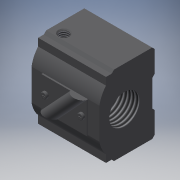
# Autodesk Inventor part: BNT 1605-2.6 Nut
Saved by Autodesk Inventor 2016 (Build 200138000, 138)
## iProperties
Category: PARTsolutions
Company: THK
Created: 2017-05-16
Part Number: BNT 1605-2.6 Nut
Catalog Web Link: www.cadenas.de
Description: BNT Nut-
Vendor: THK
Document SubType Name: Modeling
Designer: psAdmin
Manufacturer: THK
Mass: 33.6267 g
Surface Area: 94.5297 cm^2
Volume: 33.6267 cm^3
Density: 1 g/cm^3
Material: Generic
Appearance: PSOLRGB-192-192-192
PSOL_IDENT_0: {$CADENAS_DATA\23d-libs\thk\fed_screw\ball_screw\ball_screw\standard_lead_rbs\bnt\bnt_nut.prj},175 {
PSOL_IDENT_1: VTYP=3D},{NB=BNT 1605-2.6 Nut},{LINA=BNT 1605-2.6 Nut},{NN=BNT Nut},{DATE=08.03.2011 04:19:39},{GEOM
PSOL_IDENT_2: DATE=23.11.2007 13:11:00},{VERSION=},{LINEID=10},{LINESUBID=-1},{WBVAR=}  {NB=BNT 1605-2.6 Nut},{LIN
PSOL_IDENT_3: A=BNT 1605-2.6 Nut},{KT=DUMMY},{MN=BNT 1605-2.6},{L=36.000},{EL=1711.000},{W=42.000},{F=16.000},{B=3
PSOL_IDENT_4: 2.000},{C=22.000},{W1=21.000},{T=21.500},{M=32.500},{NDM=5.000},{KDM=4.134},{SL=8.000},{N1=6.000},{N
PSOL_IDENT_5: 2=2.000},{A=6.000},{M1=29.250},{X1=1.260},{X2=3.000},{R1=15.320},{X3=3.990},{ANG=47.0},{DK=3.200},{Y=
PSOL_IDENT_6: 0.740},{X4=0.300},{SD=16},{SL2=7.000},{Y2=11.700}
NN: BNT Nut
NB: BNT 1605-2.6 Nut
NBSYN: $MN. Nut
LINA: BNT 1605-2.6 Nut
MN: BNT 1605-2.6
L: 36.000
EL: 1711.000
W: 42.000
F: 16.000
B: 32.000
C: 22.000
W1: 21.000
T: 21.500
M: 32.500
NDM: 5.000
KDM: 4.134
SL: 8.000
N1: 6.000
N2: 2.000
A: 6.000
M1: 29.250
X1: 1.260
X2: 3.000
R1: 15.320
X3: 3.990
ANG: 47.0
DK: 3.200
Y: 0.740
X4: 0.300
SD: 16
SL2: 7.000
Y2: 11.700
SUPPLIER: THK
ARTICLENO: BNT 1605-2.6 Nut
BOMINFO: BNT 1605-2.6 Nut
CREATOR: CADENAS GmbH
Title: BNT 1605-2.6 Nut
Author: Cadenas PARTsolutions
Autodesk Inventor part; units mm, degrees
sketch "Sketch_1" plane through (0, 0, 0) normal (1, 0, 0) x (0, 1, 0)
  line L0 (14.74, 21) -> (-5.5, 21)
  line L1 (-5.5, 21) -> (-6.76, 19.74)
  line L2 (-6.76, 19.74) -> (-9.76, 19.74)
  line L3 (-9.76, 19.74) -> (-9.76, 15.75)
  arc A0 (-9.76, 15.75) -> (-13.25, 8.26) centre (1.867, 5.7743) ccw
  line L4 (-13.25, 8.26) -> (-13.25, -8.26)
  arc A1 (-13.25, -8.26) -> (-9.76, -15.75) centre (1.867, -5.7743) ccw
  line L5 (-9.76, -15.75) -> (-9.76, -19.74)
  line L6 (-9.76, -19.74) -> (-6.76, -19.74)
  line L7 (-6.76, -19.74) -> (-5.5, -21)
  line L8 (-5.5, -21) -> (14.74, -21)
  line L9 (14.74, -21) -> (16, -19.74)
  line L10 (16, -19.74) -> (16, -8.26)
  line L11 (16, -8.26) -> (14.74, -7)
  line L12 (14.74, -7) -> (14.74, 7)
  line L13 (14.74, 7) -> (16, 8.26)
  line L14 (16, 8.26) -> (16, 19.74)
  line L15 (16, 19.74) -> (14.74, 21)
  circle A2 centre (0, 0) radius 8
  constraints: 32 end point, 4 point on circle, 3 centre point
extrude "Extrusion1" add sketch "Sketch_1" along normal blind 36
sketch "Sketch_2" plane through (18, 0, 0) normal (0.682, 0, 0.7314) x (0.7314, 0, -0.682)
  line L0 (-18, -14.0625) -> (-3.1468, -14.0625)
  arc A0 (-3.1468, -14.0625) -> (3.1468, -14.0625) centre (0, -13.25) ccw
  line L1 (3.1468, -14.0625) -> (18, -14.0625)
  line L2 (18, -14.0625) -> (18, -13.25)
  line L3 (18, -13.25) -> (-18, -13.25)
  line L4 (-18, -13.25) -> (-18, -14.0625)
  constraints: 10 end point, 2 point on circle, 1 centre point
extrude "Extrusion2" add sketch "Sketch_2" along normal mid plane 36
sketch "Sketch_3" plane through (0, -13.25, 0) normal (0, 1, 0) x (1, 0, 0)
  line L0 (-18, -36) -> (54, -36)
  line L1 (54, -36) -> (54, 36)
  line L2 (54, 36) -> (-18, 36)
  line L3 (-18, 36) -> (-18, -36)
  line L4 (6, -8.26) -> (30, -8.26)
  line L5 (30, -8.26) -> (30, 8.26)
  line L6 (30, 8.26) -> (6, 8.26)
  line L7 (6, 8.26) -> (6, -8.26)
  constraints: 16 end point
extrude "Extrusion3" cut sketch "Sketch_3" against normal blind 3.25
sketch "Sketch_4" plane through (0, 0, 0) normal (0, 0, 1) x (1, 0, 0)
  line L0 (8.34, -15.3425) -> (8.34, -14.0625)
  line L1 (8.34, -14.0625) -> (9.94, -14.0625)
  line L2 (9.94, -14.0625) -> (9.94, -15.0225)
  arc A0 (9.62, -15.3425) -> (9.94, -15.0225) centre (9.62, -15.0225) ccw
  line L3 (9.62, -15.3425) -> (8.34, -15.3425)
  line L4 (8.34, -15.3425) -> (8.34, -14.0625)
  constraints: 10 end point, 2 point on circle, 1 centre point
revolve "Revolution1" add sketch "Sketch_4" angle 360 about axis through (8.34, -15.3425, 0) along (0, -1, 0)
sketch "Sketch_5" plane through (0, 0, 0) normal (0, 0, 1) x (1, 0, 0)
  line L0 (27.66, -15.3425) -> (27.66, -14.0625)
  line L1 (27.66, -14.0625) -> (29.26, -14.0625)
  line L2 (29.26, -14.0625) -> (29.26, -15.0225)
  arc A0 (28.94, -15.3425) -> (29.26, -15.0225) centre (28.94, -15.0225) ccw
  line L3 (28.94, -15.3425) -> (27.66, -15.3425)
  line L4 (27.66, -15.3425) -> (27.66, -14.0625)
  constraints: 10 end point, 2 point on circle, 1 centre point
revolve "Revolution2" add sketch "Sketch_5" angle 360 about axis through (27.66, -15.3425, 0) along (0, -1, 0)
sketch "Sketch_6" plane through (0, -15.3425, 0) normal (0, 1, 0) x (1, 0, 0)
  line L0 (26.86, 0.15) -> (26.86, -0.15)
  line L1 (26.86, -0.15) -> (27.51, -0.15)
  line L2 (27.51, -0.15) -> (27.51, -0.8)
  line L3 (27.51, -0.8) -> (27.81, -0.8)
  line L4 (27.81, -0.8) -> (27.81, -0.15)
  line L5 (27.81, -0.15) -> (28.46, -0.15)
  line L6 (28.46, -0.15) -> (28.46, 0.15)
  line L7 (28.46, 0.15) -> (27.81, 0.15)
  line L8 (27.81, 0.15) -> (27.81, 0.8)
  line L9 (27.81, 0.8) -> (27.51, 0.8)
  line L10 (27.51, 0.8) -> (27.51, 0.15)
  line L11 (27.51, 0.15) -> (26.86, 0.15)
  constraints: 24 end point
extrude "Extrusion4" cut sketch "Sketch_6" along normal blind 0.64
sketch "Sketch_7" plane through (0, -15.3425, 0) normal (0, 1, 0) x (1, 0, 0)
  line L0 (7.54, 0.15) -> (7.54, -0.15)
  line L1 (7.54, -0.15) -> (8.19, -0.15)
  line L2 (8.19, -0.15) -> (8.19, -0.8)
  line L3 (8.19, -0.8) -> (8.49, -0.8)
  line L4 (8.49, -0.8) -> (8.49, -0.15)
  line L5 (8.49, -0.15) -> (9.14, -0.15)
  line L6 (9.14, -0.15) -> (9.14, 0.15)
  line L7 (9.14, 0.15) -> (8.49, 0.15)
  line L8 (8.49, 0.15) -> (8.49, 0.8)
  line L9 (8.49, 0.8) -> (8.19, 0.8)
  line L10 (8.19, 0.8) -> (8.19, 0.15)
  line L11 (8.19, 0.15) -> (7.54, 0.15)
  constraints: 24 end point
extrude "Extrusion5" cut sketch "Sketch_7" along normal blind 0.64
sketch "Sketch8" plane through (0, -5.5, 21) normal (0, 0, 1) x (1, 0, 0)
  point P0 (6, 3.5)
hole "Hole1" at (6, -2, 21) direction (0, 0, -1) diameter 4.917 depth 13.5806 tip angle 120 countersink diameter 6 countersink angle 90 thread size "M6x1" class "6H" standard "ISO Metric profile"
sketch "Sketch9" plane through (0, 16, -8.26) normal (0, 1, 0) x (1, 0, 0)
  point P0 (7, 7.74)
hole "Hole2" at (7, 16, -16) direction (0, -1, 0) diameter 4.134 depth 10.5066 tip angle 120 countersink diameter 5 countersink angle 90 thread size "M5x0.8" class "6H" standard "ISO Metric profile"
pattern_linear "Rectangular Pattern1" count 2 spacing 22 along (1, 0, 0) count 2 spacing 32 along (0, 0, 1) of "Hole2"
ref_plane "bnt_nut_1_XY" through (0, 0, 0) normal (1, 0, 0) x (0, 0, -1)
ref_plane "bnt_nut_1_YZ" through (0, 0, 0) normal (0, 0, -1) x (0, 1, 0)
ref_plane "bnt_nut_1_ZX" through (0, 0, 0) normal (0, 1, 0) x (1, 0, 0)
thread "Thread1" size "M16x2" class "6H" standard "ISO Metric profile" full length
body "Solid1"
